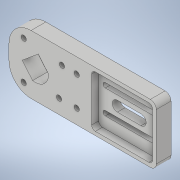
# Autodesk Inventor part: Skateboard Motor Bracket
Saved by Autodesk Inventor 2020 (Build 240168000, 168)
## iProperties
Created: 2018-10-08
Part Number: Skateboard Motor Bracket
Material: Generic
Document SubType Name: Modeling
Designer: LSabe
Density: 1 g/cm^3
Appearance: Default
Author: LSabe
Autodesk Inventor part; units mm, degrees
ref_plane "YZ Plane" through (0, 0, 0) normal (1, 0, 0) x (0, 1, 0)
ref_plane "XZ Plane" through (0, 0, 0) normal (0, 1, 0) x (-1, 0, 0)
ref_plane "XY Plane" through (0, 0, 0) normal (0, 0, 1) x (1, 0, 0)
sketch "Sketch1" plane through (0, 0, 0) normal (0, 0, 1) x (1, 0, 0)
  line L0 (0, 0) -> (127, 0)
  line L1 (127, 0) -> (127, 50.8)
  line L2 (127, 50.8) -> (0, 50.8)
  line L3 (0, 50.8) -> (0, 0)
  line L4 (0, 25.4) -> (6.35, 25.4)
  line L5 (0, 25.4) -> (6.35, 25.4) construction
  line L6 (6.35, 25.4) -> (15.367, 25.4)
  line L7 (127, 25.4) -> (120.65, 25.4)
  line L8 (127, 25.4) -> (133.35, 25.4) construction
  line L9 (15.367, 25.4) -> (15.367, 34.417)
  line L10 (15.367, 25.4) -> (24.384, 25.4) construction
  line L11 (15.367, 25.4) -> (15.367, 16.383)
  line L12 (20.3793, 14.0457) -> (11.3996, 24.7474)
  line L13 (24.8663, 36.7543) -> (33.846, 26.0526) construction
  line L14 (11.3996, 24.7474) -> (25.2144, 36.3394)
  line L15 (25.2144, 36.3394) -> (34.1942, 25.6377)
  line L16 (15.367, 25.4) -> (11.049, 25.4)
  arc A0 (20.3793, 14.0457) -> (34.1942, 25.6377) centre (22.6228, 25.4) ccw
  line L17 (120.65, 25.4) -> (131.064, 25.4) construction
  line L18 (22.6228, 25.4) -> (107.7128, 25.4)
  line L19 (22.6228, 25.4) -> (107.7128, 25.4) construction
  line L20 (22.6228, 25.4) -> (87.3928, 25.4)
  line L21 (22.6228, 25.4) -> (87.3928, 25.4) construction
  line L22 (87.3928, 25.4) -> (107.7128, 25.4)
  line L23 (107.7128, 25.4) -> (87.3928, 25.4) construction
  line L24 (107.7128, 29.845) -> (87.3928, 29.845)
  line L25 (87.3928, 20.955) -> (107.7128, 20.955)
  arc A1 (107.7128, 20.955) -> (107.7128, 29.845) centre (107.7128, 25.4) ccw
  arc A2 (87.3928, 29.845) -> (87.3928, 20.955) centre (87.3928, 25.4) ccw
  line L26 (107.7128, 25.4) -> (107.7128, 35.814)
  line L27 (107.7128, 25.4) -> (118.1268, 25.4) construction
  line L28 (107.7128, 35.814) -> (118.1268, 35.814)
  line L29 (107.7128, 35.814) -> (118.1268, 35.814) construction
  line L30 (107.7128, 14.986) -> (118.1268, 14.986)
  line L31 (97.5528, 25.4) -> (97.5528, 27.2043)
  line L32 (87.3928, 35.814) -> (76.9788, 35.814)
  line L33 (87.3928, 35.814) -> (76.9788, 35.814) construction
  line L34 (87.3928, 14.986) -> (76.9788, 14.986)
  line L35 (97.5528, 35.814) -> (97.5528, 14.986)
  line L36 (97.5528, 35.814) -> (118.3808, 35.814) construction
  line L37 (118.1268, 35.814) -> (76.9788, 35.814) construction
  line L38 (118.1268, 37.846) -> (76.9788, 37.846)
  line L39 (76.9788, 33.782) -> (118.1268, 33.782)
  arc A3 (118.1268, 33.782) -> (118.1268, 37.846) centre (118.1268, 35.814) ccw
  arc A4 (76.9788, 37.846) -> (76.9788, 33.782) centre (76.9788, 35.814) ccw
  line L40 (118.1268, 14.986) -> (76.9788, 14.986) construction
  line L41 (118.1268, 17.018) -> (76.9788, 17.018)
  line L42 (76.9788, 12.954) -> (118.1268, 12.954)
  arc A5 (118.1268, 12.954) -> (118.1268, 17.018) centre (118.1268, 14.986) ccw
  arc A6 (76.9788, 17.018) -> (76.9788, 12.954) centre (76.9788, 14.986) ccw
  dimension "d1" = 127
  dimension "d2" = 50.8
  dimension "d3" = 6.35
  dimension "d4" = 0
  dimension "d5" = 9.017
  dimension "d6" = 180
  dimension "d7" = 6.35
  dimension "d8" = 180
  dimension "d11" = 9.017
  dimension "d12" = 90
  dimension "d13" = 13.97
  dimension "d14" = 180
  dimension "d15" = 4.318
  dimension "d18" = 85.09
  dimension "d20" = 64.77
  dimension "d22" = 8.89
  dimension "d23" = 10.414
  dimension "d24" = 90
  dimension "d25" = 10.414
  dimension "d26" = 0
  dimension "d27" = 90
  dimension "d28" = 4.064
  dimension "d29" = 4.064
  dimension "d41" = 20.828
  constraints: 92 end point, 15 horizontal, 14 point on circle, 12 tangent, 9 equal length, 7 centre point, 7 symmetric about line, 6 midpoint, 6 parallel, 3 collinear, 3 perpendicular, 3 vertical, 1 point on line
  measures "d1" distance of L2.end L1.end
  measures "d2" distance of L1.end L0.end
  measures "d3" distance of L4.start L4.end
  measures "d4" distance between parallel lines of L4 L5
  measures "d5" distance of L4.end L6.end
  measures "d6" angle of L6 L4
  measures "d7" distance of L7.start L7.end
  measures "d8" angle of L7 L8
  measures "d11" distance of L9.end L6.end
  measures "d12" angle of L10 L9
  measures "d13" distance of L12.start L12.end
  measures "d14" angle of L12 L13
  measures "d15" distance of L6.end L16.end
  measures "d18" distance of L18.start L18.end
  measures "d20" distance of L20.start L20.end
  measures "d22" diameter of A2
  measures "d23" distance of L23.start L26.end
  measures "d24" angle of L27 L26
  measures "d25" distance of L26.end L28.end
  measures "d26" distance between parallel lines of L28 L29
  measures "d27" angle of L35 L36
  measures "d28" diameter of A4
  measures "d29" diameter of A6
  measures "d41" distance of L35.start L35.end
extrude "Extrusion1" add sketch "Sketch1" along normal blind 12.7 contours L3 L2 L1 L0 | L35 L39 L26 L24
sketch "Sketch2" plane through (0, 0, 12.7) normal (0, 0, 1) x (1, 0, 0)
  line L0 (127, 0) -> (127, 50.8)
  line L1 (71.2806, 47.625) -> (123.825, 47.625)
  line L2 (123.825, 47.625) -> (123.825, 3.175)
  line L3 (123.825, 3.175) -> (71.2806, 3.175)
  line L4 (71.2806, 47.625) -> (71.2806, 3.175)
  line L5 (127, 50.8) -> (68.1056, 50.8)
  line L6 (68.1056, 0) -> (127, 0)
  line L7 (68.1056, 50.8) -> (68.1056, 0)
  point P0 (0, 0)
  constraints: 16 end point, 2 parallel, 1 horizontal
extrude "Extrusion2" cut sketch "Sketch2" against normal blind 6.096 contours L1 L2 L3 L4
fillet "Fillet1" radius 5.08 2 edges at (127, 0, 6.35) (127, 50.8, 6.35)
fillet "Fillet2" radius 3.175 4 edges at (123.825, 47.625, 9.652) (71.2806, 47.625, 9.652) (71.2806, 3.175, 9.652) (123.825, 3.175, 9.652)
sketch "Sketch3" plane through (0, 0, 12.7) normal (0, 0, 1) x (1, 0, 0)
  line L0 (121.92, 50.8) -> (0, 50.8) projected
  line L1 (60.96, 50.8) -> (60.96, -0.3735)
  line L2 (60.96, 50.8) -> (112.1335, 50.8) construction
  line L3 (60.96, -0.3735) -> (60.96, 12.3265)
  line L4 (60.96, 12.3265) -> (43.18, 12.3265)
  circle A0 centre (43.18, 12.3265) radius 2.286
  circle A1 centre (45.72, 38.1) radius 2.286
  line L5 (0, 50.8) -> (0, 0) projected
  line L6 (0, 25.4) -> (12.7, 25.4)
  line L7 (0, 25.4) -> (12.7, 25.4) construction
  line L8 (12.7, 25.4) -> (12.7, 8.89)
  line L9 (12.7, 25.4) -> (29.21, 25.4) construction
  circle A2 centre (12.7, 8.89) radius 2.286
  circle A3 centre (12.7, 41.91) radius 2.286
  line L10 (60.96, 25.2132) -> (58.42, 25.2132)
  line L11 (60.96, 25.2132) -> (63.5, 25.2132) construction
  line L12 (58.42, 25.2132) -> (58.42, 37.9132)
  circle A4 centre (58.42, 37.9132) radius 2.286
  circle A5 centre (58.42, 12.5132) radius 2.286
  point P0 (3.175, 50.8)
  point P1 (0, 47.625)
  point P2 (0, 3.175)
  dimension "d42" = 90
  dimension "d43" = 12.7
  dimension "d44" = 0
  dimension "d45" = 17.78
  dimension "d46" = 4.572
  dimension "d47" = 12.7
  dimension "d48" = 0
  dimension "d49" = 16.51
  dimension "d50" = 90
  dimension "d51" = 4.572
  dimension "d52" = 2.54
  dimension "d53" = 180
  dimension "d54" = 4.572
  constraints: 22 end point, 7 horizontal, 6 centre point, 4 equal length, 3 coincident, 3 midpoint, 2 symmetric about line, 2 vertical, 1 collinear, 2 other
  measures "d42" angle of L1 L2
  measures "d43" distance of L1.end L3.end
  measures "d44" distance between parallel lines of L1 L3
  measures "d45" distance of L3.end L4.end
  measures "d46" diameter of A0
  measures "d47" distance of L6.start L6.end
  measures "d48" distance between parallel lines of L6 L7
  measures "d49" distance of L7.end L8.end
  measures "d50" angle of L8 L9
  measures "d51" diameter of A2
  measures "d52" distance of L10.start L10.end
  measures "d53" angle of L10 L11
  measures "d54" diameter of A4
extrude "Extrusion3" cut sketch "Sketch3" against normal blind 25.4
fillet "Fillet3" radius 19.05 2 edges at (0, 50.8, 6.35) (0, 0, 6.35)
body "Solid1"
